Sprossengriff (Autodesk Fusion 360 design; units mm, degrees)
Autodesk Fusion 360 part; units mm, degrees
sketch "Sketch1" plane through (0, 0, 0) normal (0, 0, 1) x (1, 0, 0)
  circle A0 centre (0, 0) radius 1.75
  circle A1 centre (18.5, 0) radius 1.75
  line L0 (-20, 7) -> (24.5, 7)
  line L1 (24.5, 7) -> (24.5, -7)
  line L2 (24.5, -7) -> (-20, -7)
  line L3 (-20, -7) -> (-20, 7)
  arc A2 (-20, -7) -> (-107.1054, -25.8531) centre (-20, -217.6501) ccw
  arc A3 (-20, -7) -> (-20, 7) centre (-20, 0) ccw
  arc A4 (-20, 7) -> (-112.8946, -13.106) centre (-20, -217.6501) ccw
  arc A5 (-112.8946, -13.106) -> (-107.1054, -25.8531) centre (-110, -19.4796) ccw
  arc A6 (-20, 0) -> (-110, -19.4796) centre (-20, -217.6501) ccw construction
  dimension "d1" = 3.5
  dimension "d2" = 3.5
  dimension "d3" = 18.5
  dimension "d4" = 6
  dimension "d5" = 7
  dimension "d6" = 7
  dimension "d7" = 20
  constraint coincident A0.centre origin
  constraint horizontal L0
  constraint vertical L1
  constraint horizontal L2
  constraint vertical L3
  constraint tangent A2 A3
  constraint tangent A3 A4
  constraint tangent A4 A5
  constraint tangent A2 A5
  constraint midpoint L3 A3.centre
  measures "d1" diameter of A0
  measures "d2" diameter of A1
  measures "d3" distance of A0.centre A1.centre
  measures "d4" distance of A1.centre L1
  measures "d5" distance of A1.centre L0
  measures "d6" distance of A1.centre L2
  measures "d7" distance of A0.centre L3
extrude "Extrude1" add sketch "Sketch1" along normal blind 4 contours A0 | A1 | L3 A3 | L0 L1 L2 A3 | L3 A2 A4 A5
extrude "Extrude2" add sketch "Sketch1" along normal blind 19 contours L3 A2 A4 A5
extrude "Extrude3" add sketch "Sketch1" along normal blind 4 from surface at 15 contours A0 | A1 | L3 A3 | L0 L1 L2 A3 | L3 A2 A4 A5
extrude "Extrude4" cut sketch "Sketch1" along normal blind 35 contours A0
extrude "Extrude5" cut sketch "Sketch1" along normal blind 19 contours A1
fillet "Fillet1" radius 4 4 edges at (24.5, -7, 17) (24.5, -7, 2) (24.5, 7, 17) (24.5, 7, 2)
fillet "Fillet2" radius 1.5 16 edges at (-64.5612, -11.7672, 19) (0.25, -7, 19) (23.3284, -5.8284, 19) (24.5, 0, 19) (23.3284, 5.8284, 19) (0.25, 7, 19) (-67.5228, 1.916, 19) (-116.3735, -22.3741, 19) (-64.5612, -11.7672, 0) (0.25, -7, 0) (23.3284, -5.8284, 0) (24.5, 0, 0) (23.3284, 5.8284, 0) (0.25, 7, 0) (-67.5228, 1.916, 0) (-116.3735, -22.3741, 0)
